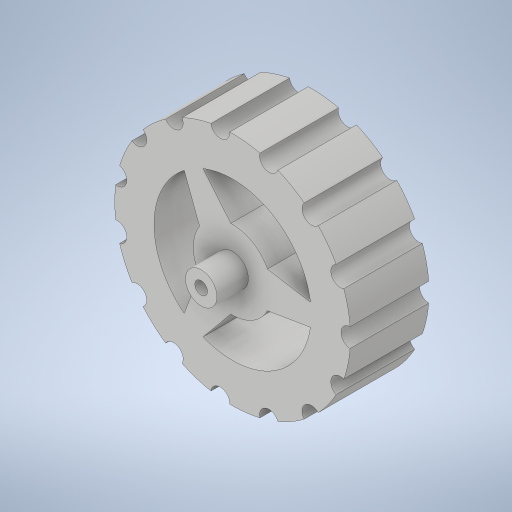
# Autodesk Inventor part: Guntas_Wheel
Saved by Autodesk Inventor 2024 (Build 280153000, 153)
## iProperties
Created: 2023-06-29
Part Number: Guntas_Wheel
Material: Generic
Document SubType Name: Modeling
Designer: gaura
Density: 1 g/cm^3
Appearance: Default
Author: gaura
Autodesk Inventor part; units mm, degrees
ref_plane "YZ Plane" through (0, 0, 0) normal (1, 0, 0) x (0, 1, 0)
ref_plane "XZ Plane" through (0, 0, 0) normal (0, 1, 0) x (-1, 0, 0)
ref_plane "XY Plane" through (0, 0, 0) normal (0, 0, 1) x (1, 0, 0)
sketch "Sketch1" plane through (0, 0, 0) normal (0, 0, 1) x (1, 0, 0)
  circle A0 centre (0, 0) radius 75
  dimension "d0" = 150
  constraints: 1 centre point, 1 coincident
  measures "d0" diameter of A0
extrude "Extrusion1" add sketch "Sketch1" along normal blind 17.5 and the other way blind 32.5
sketch "Sketch2" plane through (0, 0, 0) normal (0, 0, 1) x (1, 0, 0)
  circle A0 centre (0, 0) radius 50
  dimension "d3" = 100
  constraints: 1 centre point, 1 coincident
  measures "d3" diameter of A0
extrude "Extrusion2" cut sketch "Sketch2" along normal blind 17.5 and the other way blind 32.5
sketch "Sketch3" plane through (0, 0, 0) normal (0, 0, 1) x (1, 0, 0)
  circle A0 centre (0, 0) radius 25
  dimension "d6" = 50
  constraints: 1 centre point, 1 coincident
  measures "d6" diameter of A0
extrude "Extrusion3" add sketch "Sketch3" along normal blind 17.5 and the other way blind 32.5
sketch "Sketch5" plane through (0, 0, 17.5) normal (0, 0, 1) x (1, 0, 0)
  circle A0 centre (0, 0) radius 10
  dimension "d12" = 20
  constraints: 1 centre point, 1 coincident
  measures "d12" diameter of A0
extrude "Extrusion4" add sketch "Sketch5" along normal blind 20
sketch "Sketch6" plane through (0, 0, 37.5) normal (0, 0, 1) x (1, 0, 0)
  circle A0 centre (0, 0) radius 4
  dimension "d15" = 8
  constraints: 1 centre point, 1 coincident
  measures "d15" diameter of A0
extrude "Extrusion5" cut sketch "Sketch6" against normal blind 20
sketch "Sketch7" plane through (0, 0, 17.5) normal (0, 0, 1) x (1, 0, 0)
  circle A0 centre (0, 0) radius 75 projected
  circle A1 centre (75, 0) radius 6
  circle A2 centre (68.5159, -30.5052) radius 6
  circle A3 centre (50.1848, -55.7359) radius 6
  circle A4 centre (23.1763, -71.3292) radius 6
  circle A5 centre (-7.8396, -74.5891) radius 6
  circle A6 centre (-37.5, -64.9519) radius 6
  circle A7 centre (-60.6763, -44.0839) radius 6
  circle A8 centre (-73.3611, -15.5934) radius 6
  circle A9 centre (-73.3611, 15.5934) radius 6
  circle A10 centre (-60.6763, 44.0839) radius 6
  circle A11 centre (-37.5, 64.9519) radius 6
  circle A12 centre (-7.8396, 74.5891) radius 6
  circle A13 centre (23.1763, 71.3292) radius 6
  circle A14 centre (50.1848, 55.7359) radius 6
  circle A15 centre (68.5159, 30.5052) radius 6
  dimension "d18" = 12
  dimension "d21" = 360
  constraints: 15 centre point, 1 horizontal alignment, 32 other
  measures "d18" diameter of A1
extrude "Extrusion6" cut sketch "Sketch7" against normal up to next contours A0 A1 | A0 A1 | A15 A0 | A0 A15 | A2 A0 | A0 A2 | A14 A0 | A0 A14 | A3 A0 | A0 A3 | A13 A0 | A0 A13 | A4 A0 | A0 A4 | A12 A0 | A0 A12 | A5 A0 | A0 A5 | A11 A0 | A0 A11 | A6 A0 | A0 A6 | A10 A0 | A0 A10 | A7 A0 | A0 A7 | A9 A0 | A0 A9 | A8 A0 | A0 A8
sketch "Sketch8" plane through (0, 0, 0) normal (0, 0, 1) x (1, 0, 0)
  circle A0 centre (0, 0) radius 4 construction
  circle A1 centre (0, 0) radius 4 projected
  circle A2 centre (0, 0) radius 10 projected
  arc A3 (49.5134, -6.9587) -> (49.5134, 6.9587) centre (0, 0) ccw
  line L0 (0, 0) -> (4.4798, 14.3154) construction
  line L1 (0, 0) -> (4.4798, -14.3154) construction
  line L2 (49.5134, 6.9587) -> (10.3161, 13.4586)
  line L3 (0, 0) -> (50, 0) construction
  circle A4 centre (0, 0) radius 50 construction
  line L4 (49.5134, -6.9587) -> (10.3161, -13.4586)
  arc A5 (10.3161, -13.4586) -> (10.3161, 13.4586) centre (0, 0) ccw
  line L5 (-30.7831, -39.4005) -> (-16.8136, -2.2047)
  arc A6 (-16.8136, -2.2047) -> (6.4975, -15.6633) centre (0, 0) ccw
  line L6 (-18.7303, -46.3592) -> (6.4975, -15.6633)
  arc A7 (-30.7831, -39.4005) -> (-18.7303, -46.3592) centre (0, 0) ccw
  line L7 (-18.7303, 46.3592) -> (6.4975, 15.6633)
  arc A8 (6.4975, 15.6633) -> (-16.8136, 2.2047) centre (0, 0) ccw
  line L8 (-30.7831, 39.4005) -> (-16.8136, 2.2047)
  arc A9 (-18.7303, 46.3592) -> (-30.7831, 39.4005) centre (0, 0) ccw
  point P0 (-25, -43.3013)
  point P1 (-25, 43.3013)
  dimension "d35" = 360
  constraints: 18 end point, 14 point on circle, 6 centre point, 2 coincident, 1 symmetric about line, 34 other
extrude "Extrusion7" add sketch "Sketch8" along normal blind 17.5 and the other way blind 32.5 contours L4 A5 L2 A3 | L5 A6 L6 A7 | L7 A8 L8 A9
body "Solid1"
